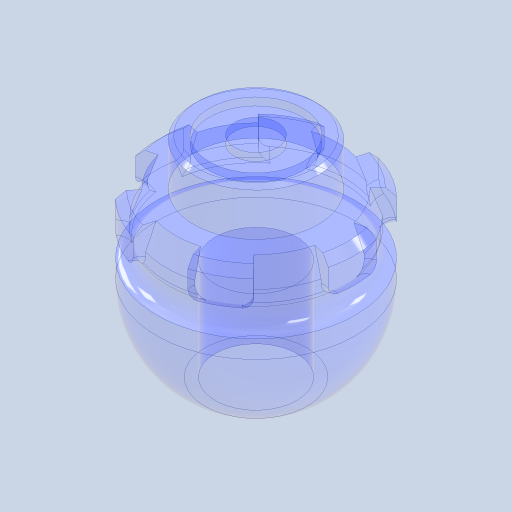
# Autodesk Inventor part: cpd_ultra-TLA100.3_0.7_p1_20230615
Saved by Autodesk Inventor 2024 (Build 280153000, 153)
## iProperties
Created: 2022-02-17
Part Number: cpd_ultra-TLA100.3_0.7_p1_20230615
Material: Generic
Document SubType Name: Modeling
Designer: to172
Density: 1 g/cm^3
Appearance: Clear - Blue
Author: to172
Autodesk Inventor part; units mm, degrees
ref_plane "YZ Plane" through (0, 0, 0) normal (1, 0, 0) x (0, 1, 0)
ref_plane "XZ Plane" through (0, 0, 0) normal (0, 1, 0) x (-1, 0, 0)
ref_plane "XY Plane" through (0, 0, 0) normal (0, 0, 1) x (1, 0, 0)
sketch "Sketch1" plane through (0, 0, 0) normal (0, 0, 1) x (1, 0, 0)
  line L0 (0, 0) -> (0, 17.8598) construction
  line L1 (0, 0) -> (17.566, 0) construction
  arc A0 (0, -6.4) -> (6.4, 0) centre (0, 0) ccw
  line L2 (0, 8) -> (0, 0)
  line L3 (0, 0) -> (0, -6.4)
  line L4 (6.4, 0) -> (6.4, 5)
  line L5 (6.4, 5) -> (4, 5)
  line L6 (4, 5) -> (4, 8)
  line L7 (0, 8) -> (1.39, 8)
  line L8 (1.39, 8) -> (1.39, 7.5)
  line L9 (1.39, 7.5) -> (3, 7.5)
  line L10 (3, 7.5) -> (3, 8)
  line L11 (3, 8) -> (4, 8)
  dimension "d1" = 12.8
  dimension "d3" = 5
  dimension "d5" = 4
  dimension "d7" = 1.39
  dimension "d8" = 3
  dimension "d9" = 3
  dimension "d10" = 0.5
  constraints: 24 end point, 6 perpendicular, 4 point on line, 2 horizontal, 2 point on circle, 2 vertical, 1 centre point, 1 coincident, 1 collinear, 1 tangent
  measures "d1" diameter of A0
  measures "d3" distance between parallel lines of L1 L5
  measures "d5" distance between parallel lines of L0 L6
  measures "d7" distance between parallel lines of L8 L0
  measures "d8" distance between parallel lines of L0 L10
  measures "d9" distance between parallel lines of L11 L5
  measures "d10" distance between parallel lines of L7 L9
revolve "Revolution1" add sketch "Sketch1" angle 360 about axis through (0, 0, 0) along (0, 1, 0)
chamfer "Chamfer1" distance 0.5 angle 45 1 edges at (-6.4, 5, 0)
chamfer "Chamfer2" distance 0.25 angle 45 1 edges at (-4, 8, 0)
sketch "Sketch2" plane through (0, 0, 0) normal (0, 1, 0) x (-1, 0, 0)
  line L0 (0, 0) -> (0, 13.854) construction
  line L1 (0, 0) -> (-16.04, 0) construction
  circle A0 centre (0, 0) radius 2.625
  dimension "d87" = 5.25
  constraints: 4 end point, 1 centre point, 1 coincident, 1 horizontal, 1 vertical
  measures "d87" diameter of A0
extrude "Extrusion1" cut sketch "Sketch2" along normal blind 1 and the other way blind 10
sketch "Sketch6" plane through (0, 0, 0) normal (0, 0, 1) x (1, 0, 0)
  line L0 (0, 0) -> (14.9996, 0) construction
  line L1 (0, 0) -> (0, -9.1498) construction
  line L2 (0, -5.5) -> (5, -5.5)
  line L3 (5, -5.5) -> (5, -6.5)
  line L4 (5, -6.5) -> (0, -6.5)
  line L5 (0, -6.5) -> (0, -5.5)
  dimension "d50" = 5.5
  dimension "d51" = 6.5
  dimension "d52" = 5
  constraints: 12 end point, 2 horizontal, 2 parallel, 1 collinear, 1 perpendicular, 1 vertical
  measures "d50" distance between parallel lines of L0 L2
  measures "d51" distance between parallel lines of L0 L4
  measures "d52" distance between parallel lines of L1 L3
revolve "Revolution5" cut sketch "Sketch6" angle 360 about axis through (0, 0, 0) along (0, -1, 0)
sketch "Sketch9" plane through (0, 0, 0) normal (1, 0, 0) x (0, 1, 0)
  line L0 (0, 0) -> (0, 9.7735) construction
  line L1 (5, 4) -> (5, -4) construction
  line L2 (5, 0) -> (5, 11.5475) construction
  line L3 (0, 0) -> (9.7899, 0) construction
  line L4 (5, 6.4) -> (0, 6.4)
  line L5 (4.5, 6.4) -> (0, 6.4) construction
  circle A0 centre (2, 6.4) radius 0.85
  line L6 (-1.958, 0) -> (11.7479, 0) projected
  line L7 (5, 5.9) -> (5, -5.9) projected
  line L8 (2, 6.4) -> (5, 6.4)
  line L9 (5, 6.4) -> (5, 5.75)
  line L10 (5, 5.75) -> (2, 5.75)
  line L11 (2, 5.75) -> (2, 6.4)
  line L12 (3.45, 5.75) -> (5, 5.2)
  line L13 (5, 5.75) -> (5, 5.2)
  point P0 (1.15, 6.4)
  point P1 (2.85, 6.4)
  point P2 (2.5477, 5.75)
  dimension "d72" = 6.4
  dimension "d73" = 1.7
  dimension "d74" = 3
  dimension "d76" = 0.65
  dimension "d88" = 0.55
  dimension "d89" = 1.55
  constraints: 20 end point, 6 point on line, 2 horizontal, 2 parallel, 2 perpendicular, 2 vertical, 1 centre point, 1 collinear, 1 midpoint
  measures "d72" distance between parallel lines of L3 L4
  measures "d73" diameter of A0
  measures "d74" distance from line of L8.start L2
  measures "d76" distance between parallel lines of L10 L8
  measures "d88" distance from line of L12.end L10
  measures "d89" distance from line of L2 L12.start
revolve "Revolution9" cut sketch "Sketch9" angle 360 about axis through (0, -10, 0) along (0, 1, 0) contours A0 L10 L11 L4 | L11 L10 A0 L4
revolve "Revolution10" cut sketch "Sketch9" angle 32 mid plane about axis through (0, 0, 0) along (0, 1, 0) contours L9 L7 L10 A0 L4 | A0 L10 L11 L4 | L11 L10 A0 L4 | L7 L12 L10
fillet "Fillet8" radius 0.5 4 edges at (-0.8002, 2.5477, 5.694) (0.8002, 2.5477, 5.694) (-1.6653, 2.7707, 5.8075) (1.6653, 2.7707, 5.8075)
pattern_circular "Circular Pattern5" count 6 over 360 about axis through (0, -10, 0) along (0, 1, 0) of "Revolution10", "Fillet8"
body "Solid1"
